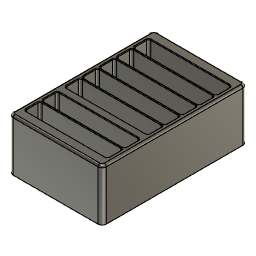
3- Caixa Organizadora (Autodesk Fusion 360 design; units mm, degrees)
Autodesk Fusion 360 part; units mm, degrees
sketch "Esboço1" plane through (0, 0, 0) normal (0, 0, 1) x (1, 0, 0)
  line L0 (20.5, 35) -> (-20.5, 35)
  line L1 (-22.5, 33) -> (-22.5, -33)
  line L2 (-20.5, -35) -> (20.5, -35)
  line L3 (22.5, -33) -> (22.5, 33)
  line L4 (22.5, 35) -> (-22.5, -35) construction
  line L5 (-22.5, 35) -> (22.5, -35) construction
  line L6 (0, 35) -> (0, 30) construction
  line L7 (-22.5, 16.9024) -> (-20, 16.9024) construction
  line L8 (-19, 30) -> (19, 30)
  line L9 (20, 29) -> (20, 23.5)
  line L10 (19, 22.5) -> (-19, 22.5)
  line L11 (-20, 23.5) -> (-20, 29)
  line L12 (0, -35) -> (0, -30) construction
  arc A0 (20, 29) -> (19, 30) centre (19, 29) ccw
  arc A1 (19, 22.5) -> (20, 23.5) centre (19, 23.5) ccw
  arc A2 (-19, 30) -> (-20, 29) centre (-19, 29) ccw
  arc A3 (-20, 23.5) -> (-19, 22.5) centre (-19, 23.5) ccw
  line L13 (19, 14.25) -> (-19, 14.25)
  arc A4 (19, 14.25) -> (20, 15.25) centre (19, 15.25) ccw
  line L14 (20, 20.75) -> (20, 15.25)
  arc A5 (20, 20.75) -> (19, 21.75) centre (19, 20.75) ccw
  line L15 (-19, 21.75) -> (19, 21.75)
  arc A6 (-19, 21.75) -> (-20, 20.75) centre (-19, 20.75) ccw
  line L16 (-20, 15.25) -> (-20, 20.75)
  arc A7 (-20, 15.25) -> (-19, 14.25) centre (-19, 15.25) ccw
  line L17 (19, 6) -> (-19, 6)
  arc A8 (19, 6) -> (20, 7) centre (19, 7) ccw
  line L18 (20, 12.5) -> (20, 7)
  arc A9 (20, 12.5) -> (19, 13.5) centre (19, 12.5) ccw
  line L19 (-19, 13.5) -> (19, 13.5)
  arc A10 (-19, 13.5) -> (-20, 12.5) centre (-19, 12.5) ccw
  line L20 (-20, 7) -> (-20, 12.5)
  arc A11 (-20, 7) -> (-19, 6) centre (-19, 7) ccw
  line L21 (19, -2.25) -> (-19, -2.25)
  arc A12 (19, -2.25) -> (20, -1.25) centre (19, -1.25) ccw
  line L22 (20, 4.25) -> (20, -1.25)
  arc A13 (20, 4.25) -> (19, 5.25) centre (19, 4.25) ccw
  line L23 (-19, 5.25) -> (19, 5.25)
  arc A14 (-19, 5.25) -> (-20, 4.25) centre (-19, 4.25) ccw
  line L24 (-20, -1.25) -> (-20, 4.25)
  arc A15 (-20, -1.25) -> (-19, -2.25) centre (-19, -1.25) ccw
  line L25 (19, -10.5) -> (-19, -10.5)
  arc A16 (19, -10.5) -> (20, -9.5) centre (19, -9.5) ccw
  line L26 (20, -4) -> (20, -9.5)
  arc A17 (20, -4) -> (19, -3) centre (19, -4) ccw
  line L27 (-19, -3) -> (19, -3)
  arc A18 (-19, -3) -> (-20, -4) centre (-19, -4) ccw
  line L28 (-20, -9.5) -> (-20, -4)
  arc A19 (-20, -9.5) -> (-19, -10.5) centre (-19, -9.5) ccw
  arc A20 (22.5, 33) -> (20.5, 35) centre (20.5, 33) ccw
  arc A21 (20.5, -35) -> (22.5, -33) centre (20.5, -33) ccw
  arc A22 (-22.5, -33) -> (-20.5, -35) centre (-20.5, -33) ccw
  arc A23 (-20.5, 35) -> (-22.5, 33) centre (-20.5, 33) ccw
  line L29 (-20, -29) -> (-20, -23.5)
  arc A24 (-19, -22.5) -> (-20, -23.5) centre (-19, -23.5) ccw
  line L30 (-19, -22.5) -> (19, -22.5)
  arc A25 (20, -23.5) -> (19, -22.5) centre (19, -23.5) ccw
  line L31 (20, -23.5) -> (20, -29)
  arc A26 (19, -30) -> (20, -29) centre (19, -29) ccw
  line L32 (19, -30) -> (-19, -30)
  arc A27 (-20, -29) -> (-19, -30) centre (-19, -29) ccw
  line L33 (-20, -20.7) -> (-20, -15.2)
  arc A28 (-19, -14.2) -> (-20, -15.2) centre (-19, -15.2) ccw
  line L34 (-19, -14.2) -> (19, -14.2)
  arc A29 (20, -15.2) -> (19, -14.2) centre (19, -15.2) ccw
  line L35 (20, -15.2) -> (20, -20.7)
  arc A30 (19, -21.7) -> (20, -20.7) centre (19, -20.7) ccw
  line L36 (19, -21.7) -> (-19, -21.7)
  arc A31 (-20, -20.7) -> (-19, -21.7) centre (-19, -20.7) ccw
  point P0 (-20, 30)
  point P1 (20, 30)
  point P2 (-20, 22.5)
  dimension "d1" = 45
  dimension "d2" = 70
  dimension "d3" = 5
  dimension "d4" = 2.5
  dimension "d5" = 40
  dimension "d6" = 7.5
  dimension "d7" = 5
  dimension "d8" = 1
  dimension "d11" = 0
  dimension "d12" = -33
  dimension "d13" = 2
  dimension "d34" = 7.5
  dimension "d35" = 7.5
  constraint horizontal L0
  constraint perpendicular L0 L1
  constraint parallel L0 L2
  constraint parallel L1 L3
  constraint coincident L4 origin
  constraint coincident L5 origin
  constraint perpendicular L0 L6
  constraint coincident L1 L7.start
  constraint perpendicular L1 L7
  constraint horizontal L8
  constraint vertical L9
  constraint horizontal L10
  constraint vertical L11
  constraint perpendicular L2 L12
  constraint coincident P1 L8
  constraint coincident P1 L9
  constraint tangent L8 A0
  constraint tangent L9 A0
  constraint tangent L9 A1
  constraint tangent L10 A1
  constraint equal A0 A1
  constraint coincident P0 L8
  constraint coincident P0 L11
  constraint tangent L8 A2
  constraint tangent L11 A2
  constraint equal A0 A2
  constraint coincident P2 L10
  constraint coincident P2 L11
  constraint tangent L10 A3
  constraint tangent L11 A3
  constraint equal A0 A3
  constraint coincident L0 L6.start
  constraint coincident L4.start L0
  constraint coincident L4.start L3
  constraint tangent L0 A20
  constraint tangent L3 A20
  constraint coincident L2 L12.start
  constraint coincident L5.end L3
  constraint coincident L5.end L2
  constraint tangent L3 A21
  constraint tangent L2 A21
  constraint equal A20 A21
  constraint coincident L4.end L2
  constraint coincident L4.end L1
  constraint tangent L2 A22
  constraint tangent L1 A22
  constraint equal A20 A22
  constraint coincident L5.start L0
  constraint coincident L5.start L1
  constraint tangent L0 A23
  constraint tangent L1 A23
  constraint equal A20 A23
  measures "d1" distance of L4.end L5.end
  measures "d2" distance of L5.start L4.end
  measures "d3" distance of L6.start L6.end
  measures "d4" distance of L7.start L7.end
  measures "d5" distance of P0 P1
  measures "d6" distance of P0 P2
  measures "d7" distance of L12.start L12.end
  measures "d8" radius of A0
  measures "d13" radius of A20
  measures "d34" distance of L30 L32
  measures "d35" distance of L34 L36
extrude "Extrusão1" add sketch "Esboço1" along normal blind 1 contours L0 L1 L2 L3 A20 A21 A22 A23 | L8 L9 L10 L11 A0 A1 A2 A3 | L13 A4 L14 A5 L15 A6 L16 A7 | L17 A8 L18 A9 L19 A10 L20 A11 | L21 A12 L22 A13 L23 A14 L24 A15 | L25 A16 L26 A17 L27 A18 L28 A19 | L29 A24 L30 A25 L31 A26 L32 A27 | L33 A28 L34 A29 L35 A30 L36 A31
extrude "Extrusão2" add sketch "Esboço1" along normal blind 25 contours L0 L1 L2 L3 A20 A21 A22 A23 | L29 A24 L30 A25 L31 A26 L32 A27 | L33 A28 L34 A29 L35 A30 L36 A31
fillet "Arredondamento1" radius 1 8 edges at (-22.5, 0, 25) (-21.9142, -34.4142, 25) (0, -35, 25) (21.9142, -34.4142, 25) (22.5, 0, 25) (21.9142, 34.4142, 25) (0, 35, 25) (-21.9142, 34.4142, 25)
fillet "Arredondamento2" radius 0.3 40 edges at (20, 26.25, 25) (19.7071, 22.7929, 25) (0, 22.5, 25) (-19.7071, 22.7929, 25) (-20, 26.25, 25) (-19.7071, 29.7071, 25) (0, 30, 25) (19.7071, 29.7071, 25) (20, 18, 25) (19.7071, 14.5429, 25) (0, 14.25, 25) (-19.7071, 14.5429, 25) (-20, 18, 25) (-19.7071, 21.4571, 25) (0, 21.75, 25) (19.7071, 21.4571, 25) (20, 9.75, 25) (19.7071, 6.2929, 25) (0, 6, 25) (-19.7071, 6.2929, 25) (-20, 9.75, 25) (-19.7071, 13.2071, 25) (0, 13.5, 25) (19.7071, 13.2071, 25) (20, 1.5, 25) (19.7071, -1.9571, 25) (0, -2.25, 25) (-19.7071, -1.9571, 25) (-20, 1.5, 25) (-19.7071, 4.9571, 25) (0, 5.25, 25) (19.7071, 4.9571, 25) (20, -6.75, 25) (19.7071, -10.2071, 25) (0, -10.5, 25) (-19.7071, -10.2071, 25) (-20, -6.75, 25) (-19.7071, -3.2929, 25) (0, -3, 25) (19.7071, -3.2929, 25)
chamfer "Chanfro1" distance 1 angle 45 8 edges at (0, -3, 1) (-19.7071, -3.2929, 1) (-20, -6.75, 1) (-19.7071, -10.2071, 1) (0, -10.5, 1) (19.7071, -10.2071, 1) (20, -6.75, 1) (19.7071, -3.2929, 1)
chamfer "Chanfro2" distance 1 angle 45 32 edges at (0, 5.25, 1) (-19.7071, 4.9571, 1) (-20, 1.5, 1) (-19.7071, -1.9571, 1) (0, -2.25, 1) (19.7071, -1.9571, 1) (20, 1.5, 1) (19.7071, 4.9571, 1) (0, 13.5, 1) (-19.7071, 13.2071, 1) (-20, 9.75, 1) (-19.7071, 6.2929, 1) (0, 6, 1) (19.7071, 6.2929, 1) (20, 9.75, 1) (19.7071, 13.2071, 1) (0, 21.75, 1) (-19.7071, 21.4571, 1) (-20, 18, 1) (-19.7071, 14.5429, 1) (0, 14.25, 1) (19.7071, 14.5429, 1) (20, 18, 1) (19.7071, 21.4571, 1) (0, 30, 1) (-19.7071, 29.7071, 1) (-20, 26.25, 1) (-19.7071, 22.7929, 1) (0, 22.5, 1) (19.7071, 22.7929, 1) (20, 26.25, 1) (19.7071, 29.7071, 1)
extrude "Extrusão3" cut sketch "Esboço1" along normal blind 24 from surface at 1 contours L29 A24 L30 A25 L31 A26 L32 A27 | L33 A28 L34 A29 L35 A30 L36 A31
fillet "Arredondamento3" radius 0.3 16 edges at (20, -17.95, 25) (19.7071, -21.4071, 25) (0, -21.7, 25) (-19.7071, -21.4071, 25) (-20, -17.95, 25) (-19.7071, -14.4929, 25) (0, -14.2, 25) (19.7071, -14.4929, 25) (20, -26.25, 25) (19.7071, -29.7071, 25) (0, -30, 25) (-19.7071, -29.7071, 25) (-20, -26.25, 25) (-19.7071, -22.7929, 25) (0, -22.5, 25) (19.7071, -22.7929, 25)
chamfer "Chanfro3" distance 1 angle 45 16 edges at (0, -14.2, 1) (19.7071, -14.4929, 1) (20, -17.95, 1) (19.7071, -21.4071, 1) (0, -21.7, 1) (-19.7071, -21.4071, 1) (-20, -17.95, 1) (-19.7071, -14.4929, 1) (0, -22.5, 1) (19.7071, -22.7929, 1) (20, -26.25, 1) (19.7071, -29.7071, 1) (0, -30, 1) (-19.7071, -29.7071, 1) (-20, -26.25, 1) (-19.7071, -22.7929, 1)
